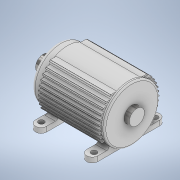
# Autodesk Inventor part: DC motor
Saved by Autodesk Inventor 2021 (Build 250183000, 183)
## iProperties
Created: 2021-07-01
Part Number: DC motor
Material: Generic
Document SubType Name: Modeling
Designer: almas
Density: 1 g/cm^3
Appearance: Default
Author: almas
Autodesk Inventor part; units mm, degrees
ref_plane "YZ Plane" through (0, 0, 0) normal (1, 0, 0) x (0, 1, 0)
ref_plane "XZ Plane" through (0, 0, 0) normal (0, 1, 0) x (-1, 0, 0)
sketch "Sketch1" plane through (0, 0, 0) normal (0, 0, 1) x (1, 0, 0)
  line L0 (0, 15.5) -> (0, 44)
  line L1 (6, 50) -> (20, 50)
  line L2 (20, 50) -> (20, 52)
  line L3 (20, 52) -> (140, 52)
  arc A0 (6, 50) -> (0, 44) centre (6, 44) ccw
  line L4 (0, 0) -> (73.0939, 0) construction
  line L5 (-1.7761, 15.5) -> (-1.7761, 44)
  arc A1 (6, 51.7761) -> (-1.7761, 44) centre (6, 44) ccw
  line L6 (6, 51.7761) -> (18.2239, 51.7761)
  line L7 (18.2239, 51.7761) -> (18.2239, 53.7761)
  line L8 (18.2239, 53.7761) -> (140, 53.7761)
  line L9 (-1.7761, 15.5) -> (0, 15.5)
  line L10 (140, 53.7761) -> (140, 52)
  point P0 (0, 50)
  dimension "d0" = 0
  dimension "d1" = 15.5
  dimension "d2" = 50
  dimension "d3" = 52
  dimension "d4" = 20
  dimension "d5" = 140
  dimension "d6" = 6
  constraints: 22 end point, 8 perpendicular, 4 point on circle, 2 centre point, 2 point on line, 2 tangent, 1 horizontal, 1 vertical, 4 other
  measures "d0" horizontal distance of L4.start L0.start
  measures "d1" distance of L4.start L0.start
  measures "d2" distance of L4.start point (0, 50)
  measures "d3" vertical distance of L4.start L2.end
  measures "d4" horizontal distance of L4.start L1.end
  measures "d5" horizontal distance of L4.start L3.end
  measures "d6" radius of A0
revolve "Revolution1" add sketch "Sketch1" angle 360 about axis through (0, 0, 0) along (1, 0, 0)
sketch "Sketch2" plane through (140, 0, 0) normal (1, 0, 0) x (0, 0, -1)
  line L0 (72.5, -43.7761) -> (72.5, -53.7761)
  line L1 (72.5, -53.7761) -> (-72.5, -53.7761)
  line L2 (-72.5, -53.7761) -> (-72.5, -43.7761)
  circle A0 centre (0, 0) radius 53.7761 projected
  circle A1 centre (0, 0) radius 52 projected
  line L3 (-72.5, -43.7761) -> (-28.0651, -43.7761)
  line L4 (28.0651, -43.7761) -> (72.5, -43.7761)
  point P0 (0, -53.7761)
  point P1 (-31.2334, -43.7761)
  point P2 (31.2334, -43.7761)
  dimension "d8" = 10
  dimension "d9" = 145
  dimension "d10" = 72.5
  constraints: 10 end point, 3 parallel, 2 horizontal, 2 perpendicular, 2 point on circle, 1 tangent
  measures "d8" distance of L0.start L0.end
  measures "d9" distance of L2.end L0.start
  measures "d10" horizontal distance of point (0, 0) L0.end
extrude "Extrusion1" add sketch "Sketch2" against normal blind 22 contours L0 L1 A0 L4 | L1 L2 L3 A0
fillet "Fillet1" radius 11 4 edges at (118, -48.7761, 72.5) (140, -48.7761, 72.5) (118, -48.7761, -72.5) (140, -48.7761, -72.5)
fillet "Fillet2" radius 5 2 edges at (129, -43.7761, 31.2334) (129, -43.7761, -31.2334)
sketch "Sketch3" plane through (129, -43.7761, 61.5) normal (0, 1, 0) x (1, 0, 0)
  point P0 (-129, 61.5)
  point P1 (1.5019, 2.0437)
  point P2 (1.8044, 122.9196)
hole "Hole1" at (130.5019, -43.7761, 59.4563) at (130.8044, -43.7761, -61.4196) direction (0, -1, 0) diameter 11 end through all
ref_plane "Work Plane1" through (78.2239, 0, 0) normal (-1, 0, 0) x (0, 0, 1)
mirror "Mirror1" about plane through (78.2239, 0, 0) normal (-1, 0, 0) of "Hole1", "Fillet2", "Fillet1", "Extrusion1"
sketch "Sketch4" plane through (140, -53.7761, 61.5) normal (1, 0, 0) x (0, 0, -1)
  point P0 (61.5, 53.7761)
sketch "Sketch5" plane through (140, -53.7761, 61.5) normal (1, 0, 0) x (0, 0, -1)
  circle A0 centre (61.5, 53.7761) radius 52
  line L0 (7.893, 27.4587) -> (16.6515, 27.4587)
  line L1 (15.254, 30) -> (7.1776, 30)
  line L2 (0, 0) -> (123, 0) projected
  line L3 (61.5, 53.7761) -> (61.5, 85.5887) construction
  line L4 (61.5, 61.7761) -> (61.5, 93.5887) construction
  line L5 (11.9509, 38) -> (4.2694, 38)
  line L6 (4.7304, 35.4587) -> (12.8331, 35.4587)
  line L7 (61.5, 69.7761) -> (61.5, 101.5887) construction
  line L8 (10.0847, 46) -> (2.5784, 46)
  line L9 (2.8155, 43.4587) -> (10.5338, 43.4587)
  line L10 (61.5, 77.7761) -> (61.5, 109.5887) construction
  line L11 (9.5005, 54) -> (2.0006, 54)
  line L12 (2.0278, 51.4587) -> (9.5517, 51.4587)
  line L13 (61.5, 85.7761) -> (61.5, 117.5887) construction
  line L14 (10.1544, 62) -> (2.5035, 62)
  line L15 (2.3221, 59.4587) -> (9.8114, 59.4587)
  line L16 (61.5, 93.7761) -> (61.5, 125.5887) construction
  line L17 (12.0957, 70) -> (4.1152, 70)
  line L18 (3.715, 67.4587) -> (11.3324, 67.4587)
  line L19 (61.5, 101.7761) -> (61.5, 133.5887) construction
  line L20 (15.4869, 78) -> (6.9342, 78)
  line L21 (6.2896, 75.4587) -> (14.2362, 75.4587)
  line L22 (61.5, 109.7761) -> (61.5, 141.5887) construction
  line L23 (20.688, 86) -> (11.1627, 86)
  line L24 (10.2236, 83.4587) -> (18.804, 83.4587)
  line L25 (61.5, 117.7761) -> (61.5, 149.5887) construction
  line L26 (28.5449, 94) -> (17.2026, 94)
  line L27 (15.8673, 91.4587) -> (25.6667, 91.4587)
  line L28 (61.5, 125.7761) -> (61.5, 157.5887) construction
  line L29 (42.046, 102) -> (25.9658, 102)
  line L30 (23.9844, 99.4587) -> (36.6584, 99.4587)
  arc A1 (3.7885, 37.3632) -> (4.2533, 35.8089) centre (61.5, 53.7761) ccw
  arc A2 (2.0833, 45.4305) -> (2.3224, 43.8762) centre (61.5, 53.7761) ccw
  arc A3 (1.5006, 53.4977) -> (1.528, 51.9434) centre (61.5, 53.7761) ccw
  arc A4 (2.0077, 61.5649) -> (1.8248, 60.0106) centre (61.5, 53.7761) ccw
  arc A5 (3.633, 69.6321) -> (3.2294, 68.0778) centre (61.5, 53.7761) ccw
  arc A6 (6.4757, 77.6994) -> (5.8257, 76.1451) centre (61.5, 53.7761) ccw
  arc A7 (10.7397, 85.7666) -> (9.7928, 84.2123) centre (61.5, 53.7761) ccw
  arc A8 (16.8303, 93.8338) -> (15.4838, 92.2795) centre (61.5, 53.7761) ccw
  arc A9 (25.6672, 101.901) -> (23.6691, 100.3468) centre (61.5, 53.7761) ccw
  arc A10 (6.7211, 29.296) -> (7.4425, 27.7417) centre (61.5, 53.7761) ccw
  arc A11 (25.9658, 102) -> (25.6672, 101.901) centre (25.9658, 101.5) ccw
  arc A12 (23.6691, 100.3468) -> (23.9844, 99.4587) centre (23.9844, 99.9587) ccw
  arc A13 (17.2026, 94) -> (16.8303, 93.8338) centre (17.2026, 93.5) ccw
  arc A14 (15.4838, 92.2795) -> (15.8673, 91.4587) centre (15.8673, 91.9587) ccw
  arc A15 (11.1627, 86) -> (10.7397, 85.7666) centre (11.1627, 85.5) ccw
  arc A16 (9.7928, 84.2123) -> (10.2236, 83.4587) centre (10.2236, 83.9587) ccw
  arc A17 (6.9342, 78) -> (6.4757, 77.6994) centre (6.9342, 77.5) ccw
  arc A18 (5.8257, 76.1451) -> (6.2896, 75.4587) centre (6.2896, 75.9587) ccw
  arc A19 (3.2294, 68.0778) -> (3.715, 67.4587) centre (3.715, 67.9587) ccw
  arc A20 (4.1152, 70) -> (3.633, 69.6321) centre (4.1152, 69.5) ccw
  arc A21 (2.5035, 62) -> (2.0077, 61.5649) centre (2.5035, 61.5) ccw
  arc A22 (1.8248, 60.0106) -> (2.3221, 59.4587) centre (2.3221, 59.9587) ccw
  arc A23 (2.0006, 54) -> (1.5006, 53.4977) centre (2.0006, 53.5) ccw
  arc A24 (1.528, 51.9434) -> (2.0278, 51.4587) centre (2.0278, 51.9587) ccw
  arc A25 (2.5784, 46) -> (2.0833, 45.4305) centre (2.5784, 45.5) ccw
  arc A26 (2.3224, 43.8762) -> (2.8155, 43.4587) centre (2.8155, 43.9587) ccw
  arc A27 (4.2694, 38) -> (3.7885, 37.3632) centre (4.2694, 37.5) ccw
  arc A28 (4.2533, 35.8089) -> (4.7304, 35.4587) centre (4.7304, 35.9587) ccw
  arc A29 (7.1776, 30) -> (6.7211, 29.296) centre (7.1776, 29.5) ccw
  arc A30 (7.4425, 27.7417) -> (7.893, 27.4587) centre (7.893, 27.9587) ccw
  line L31 (115.107, 27.4587) -> (106.3485, 27.4587)
  line L32 (107.746, 30) -> (115.8224, 30)
  line L33 (111.0491, 38) -> (118.7306, 38)
  line L34 (118.2696, 35.4587) -> (110.1669, 35.4587)
  line L35 (112.9153, 46) -> (120.4216, 46)
  line L36 (120.1845, 43.4587) -> (112.4662, 43.4587)
  line L37 (113.4995, 54) -> (120.9994, 54)
  line L38 (120.9722, 51.4587) -> (113.4483, 51.4587)
  line L39 (112.8456, 62) -> (120.4965, 62)
  line L40 (120.6779, 59.4587) -> (113.1886, 59.4587)
  line L41 (110.9043, 70) -> (118.8848, 70)
  line L42 (119.285, 67.4587) -> (111.6676, 67.4587)
  line L43 (107.5131, 78) -> (116.0658, 78)
  line L44 (116.7104, 75.4587) -> (108.7638, 75.4587)
  line L45 (102.312, 86) -> (111.8373, 86)
  line L46 (112.7764, 83.4587) -> (104.196, 83.4587)
  line L47 (94.4551, 94) -> (105.7974, 94)
  line L48 (107.1327, 91.4587) -> (97.3333, 91.4587)
  line L49 (80.954, 102) -> (97.0342, 102)
  line L50 (99.0156, 99.4587) -> (86.3416, 99.4587)
  arc A31 (118.7467, 35.8089) -> (119.2115, 37.3632) centre (61.5, 53.7761) ccw
  arc A32 (120.6776, 43.8762) -> (120.9167, 45.4305) centre (61.5, 53.7761) ccw
  arc A33 (121.472, 51.9434) -> (121.4994, 53.4977) centre (61.5, 53.7761) ccw
  arc A34 (121.1752, 60.0106) -> (120.9923, 61.5649) centre (61.5, 53.7761) ccw
  arc A35 (119.7706, 68.0778) -> (119.367, 69.6321) centre (61.5, 53.7761) ccw
  arc A36 (117.1743, 76.1451) -> (116.5243, 77.6994) centre (61.5, 53.7761) ccw
  arc A37 (113.2072, 84.2123) -> (112.2603, 85.7666) centre (61.5, 53.7761) ccw
  arc A38 (107.5162, 92.2795) -> (106.1697, 93.8338) centre (61.5, 53.7761) ccw
  arc A39 (99.3309, 100.3468) -> (97.3328, 101.901) centre (61.5, 53.7761) ccw
  arc A40 (115.5575, 27.7417) -> (116.2789, 29.296) centre (61.5, 53.7761) ccw
  arc A41 (97.3328, 101.901) -> (97.0342, 102) centre (97.0342, 101.5) ccw
  arc A42 (99.0156, 99.4587) -> (99.3309, 100.3468) centre (99.0156, 99.9587) ccw
  arc A43 (106.1697, 93.8338) -> (105.7974, 94) centre (105.7974, 93.5) ccw
  arc A44 (107.1327, 91.4587) -> (107.5162, 92.2795) centre (107.1327, 91.9587) ccw
  arc A45 (112.2603, 85.7666) -> (111.8373, 86) centre (111.8373, 85.5) ccw
  arc A46 (112.7764, 83.4587) -> (113.2072, 84.2123) centre (112.7764, 83.9587) ccw
  arc A47 (116.5243, 77.6994) -> (116.0658, 78) centre (116.0658, 77.5) ccw
  arc A48 (116.7104, 75.4587) -> (117.1743, 76.1451) centre (116.7104, 75.9587) ccw
  arc A49 (119.285, 67.4587) -> (119.7706, 68.0778) centre (119.285, 67.9587) ccw
  arc A50 (119.367, 69.6321) -> (118.8848, 70) centre (118.8848, 69.5) ccw
  arc A51 (120.9923, 61.5649) -> (120.4965, 62) centre (120.4965, 61.5) ccw
  arc A52 (120.6779, 59.4587) -> (121.1752, 60.0106) centre (120.6779, 59.9587) ccw
  arc A53 (121.4994, 53.4977) -> (120.9994, 54) centre (120.9994, 53.5) ccw
  arc A54 (120.9722, 51.4587) -> (121.472, 51.9434) centre (120.9722, 51.9587) ccw
  arc A55 (120.9167, 45.4305) -> (120.4216, 46) centre (120.4216, 45.5) ccw
  arc A56 (120.1845, 43.4587) -> (120.6776, 43.8762) centre (120.1845, 43.9587) ccw
  arc A57 (119.2115, 37.3632) -> (118.7306, 38) centre (118.7306, 37.5) ccw
  arc A58 (118.2696, 35.4587) -> (118.7467, 35.8089) centre (118.2696, 35.9587) ccw
  arc A59 (116.2789, 29.296) -> (115.8224, 30) centre (115.8224, 29.5) ccw
  arc A60 (115.107, 27.4587) -> (115.5575, 27.7417) centre (115.107, 27.9587) ccw
  point P0 (7.5798, 27.4587)
  point P1 (3.6112, 38)
  point P2 (4.3645, 35.4587)
  point P3 (2.006, 46)
  point P4 (2.3937, 43.4587)
  point P5 (1.5004, 54)
  point P6 (1.5448, 51.4587)
  point P7 (2.0663, 62)
  point P8 (1.7697, 59.4587)
  point P9 (3.7351, 70)
  point P10 (3.0809, 67.4587)
  point P11 (6.6073, 78)
  point P12 (5.5548, 75.4587)
  point P13 (10.8875, 86)
  point P14 (9.3565, 83.4587)
  point P15 (16.9799, 94)
  point P16 (14.8093, 91.4587)
  point P17 (25.8005, 102)
  point P18 (22.6013, 99.4587)
  point P19 (6.4119, 30)
  point P20 (115.4202, 27.4587)
  point P21 (119.3888, 38)
  point P22 (118.6355, 35.4587)
  point P23 (120.994, 46)
  point P24 (120.6063, 43.4587)
  point P25 (121.4996, 54)
  point P26 (121.4552, 51.4587)
  point P27 (120.9337, 62)
  point P28 (121.2303, 59.4587)
  point P29 (119.2649, 70)
  point P30 (119.9191, 67.4587)
  point P31 (116.3927, 78)
  point P32 (117.4452, 75.4587)
  point P33 (112.1125, 86)
  point P34 (113.6435, 83.4587)
  point P35 (106.0201, 94)
  point P36 (108.1907, 91.4587)
  point P37 (97.1995, 102)
  point P38 (100.3987, 99.4587)
  point P39 (116.5881, 30)
  point P40 (106.3485, 27.4587)
  point P41 (80.954, 102)
  point P42 (86.3416, 99.4587)
  point P43 (108.7638, 75.4587)
  point P44 (112.8456, 62)
  point P45 (112.9153, 46)
  point P46 (113.4995, 54)
  point P47 (113.4483, 51.4587)
  point P48 (111.0491, 38)
  constraints: 160 point on circle, 100 end point, 100 symmetric about line, 60 centre point, 40 point on line, 40 tangent, 19 equal radius, 2 coincident, 1 horizontal, 1 parallel, 1 vertical, 52 other
sketch "Sketch6" plane through (140, -53.7761, 61.5) normal (1, 0, 0) x (0, 0, -1)
  point P0 (61.5, 53.7761)
extrude "Extrusion2" add sketch "Sketch5" against normal blind 120 contours A0 L37 A53 A33 A54 L38 | A0 L39 A51 A34 A52 L40 | L35 A55 A32 A56 L36 A0 | A0 L41 A50 A35 A49 L42 | L33 A57 A31 A58 L34 A0 | A0 L43 A47 A36 A48 L44 | L32 A59 A40 A60 L31 A0 | A0 L45 A45 A37 A46 L46 | L0 A30 A10 A29 L1 A0 | A0 L47 A43 A38 A44 L48 | L6 A28 A1 A27 L5 A0 | A0 L49 A41 A39 A42 L50 | L9 A26 A2 A25 L8 A0 | A0 L30 A12 A9 A11 L29 | L12 A24 A3 A23 L11 A0 | A0 L27 A14 A8 A13 L26 | L15 A22 A4 A21 L14 A0 | A0 L24 A16 A7 A15 L23 | L18 A19 A5 A20 L17 A0 | A0 L21 A18 A6 A17 L20
sketch "Sketch7" plane through (0, 0, 0) normal (0, 1, 0) x (-1, 0, 0)
  point P0 (0, 0)
sketch "Sketch8" plane through (0, 0, 0) normal (0, 1, 0) x (-1, 0, 0)
  point P0 (0, 0)
sketch "Sketch9" plane through (0, 0, 0) normal (0, 1, 0) x (-1, 0, 0)
  line L0 (-140, 23.7977) -> (-140, -23.7977) projected
  line L1 (-140, 52) -> (-140, -52) projected
  line L2 (-140, 0) -> (-146, 0)
  line L3 (-146, 0) -> (-146, -51.5658)
  line L4 (-143, -54.5658) -> (-140, -54.5658)
  line L5 (-140, -54.5658) -> (-140, 0)
  arc A0 (-146, -51.5658) -> (-143, -54.5658) centre (-143, -51.5658) ccw
  point P0 (0, 0)
  point P1 (-140, -53.7757)
  point P2 (-146, -54.5658)
  dimension "d36" = 6
  dimension "d37" = 3
  constraints: 8 end point, 2 parallel, 2 point on circle, 2 point on line, 2 tangent, 1 centre point, 1 horizontal, 1 midpoint, 1 perpendicular
  measures "d36" distance of point (-146, -54.566) L4.end
  measures "d37" radius of A0
revolve "Revolution2" add sketch "Sketch9" angle 360 about axis through (140, 0, 0) along (1, 0, 0)
sketch "Sketch10" plane through (146, 0, 0) normal (1, 0, 0) x (0, 0, -1)
  circle A0 centre (0, 0) radius 15.5
  dimension "d39" = 31
  constraints: 1 centre point, 1 coincident
  measures "d39" diameter of A0
extrude "Extrusion3" cut sketch "Sketch10" against normal blind 120
sketch "Sketch11" plane through (146, 0, 0) normal (1, 0, 0) x (0, 0, -1)
  circle A0 centre (0, 0) radius 15.5 projected
  circle A1 centre (0, 0) radius 15
  dimension "d42" = 30
  constraints: 1 centre point, 1 coincident
  measures "d42" diameter of A1
extrude "Extrusion4" add sketch "Sketch11" along normal blind 10 and the other way blind 176 contours A1
body "Solid1"
